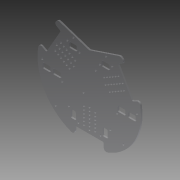
# Autodesk Inventor part: Bottom Plate
Saved by Autodesk Inventor 2015 (Build 190159000, 159)
## iProperties
Created: 2016-02-10
Part Number: Bottom Plate
Material: Polycarbonate, Clear
Document SubType Name: Modeling
Designer: James
Density: 1.2 g/cm^3
Appearance: Polycarbonate - Clear
Mass: 85.2719 g
Surface Area: 524.465 cm^2
Volume: 71.0599 cm^3
Author: James
Autodesk Inventor part; units mm, degrees
ref_plane "YZ Plane" through (0, 0, 0) normal (1, 0, 0) x (0, 1, 0)
ref_plane "XZ Plane" through (0, 0, 0) normal (0, 1, 0) x (-1, 0, 0)
ref_plane "XY Plane" through (0, 0, 0) normal (0, 0, 1) x (1, 0, 0)
sketch "Sketch1" plane through (0, 0, 0) normal (0, 1, 0) x (-1, 0, 0)
  line L0 (69.282, 40) -> (56.282, 62.5167)
  line L1 (69.282, 40) -> (82.282, 17.4833)
  circle A0 centre (63.7395, 36.8) radius 1.65
  circle A1 centre (58.2402, 33.625) radius 1.65
  circle A2 centre (52.7409, 30.45) radius 1.65
  circle A3 centre (47.2417, 27.275) radius 1.65
  circle A4 centre (41.7424, 24.1) radius 1.65
  circle A5 centre (36.2432, 20.925) radius 1.65
  circle A6 centre (30.7439, 17.75) radius 1.65
  circle A7 centre (55.6298, 44.6464) radius 1.65
  circle A8 centre (50.1305, 41.4714) radius 1.65
  circle A9 centre (44.6313, 38.2964) radius 1.65
  circle A10 centre (39.132, 35.1214) radius 1.65
  circle A11 centre (33.6327, 31.9464) radius 1.65
  circle A12 centre (28.1335, 28.7714) radius 1.65
  circle A13 centre (66.4798, 25.8536) radius 1.65
  circle A14 centre (60.9805, 22.6786) radius 1.65
  circle A15 centre (55.4813, 19.5036) radius 1.65
  circle A16 centre (49.982, 16.3286) radius 1.65
  circle A17 centre (44.4827, 13.1536) radius 1.65
  circle A18 centre (38.9835, 9.9786) radius 1.65
  line L2 (57.0141, 65.2487) -> (63.1492, 68.7908)
  line L3 (85.0141, 16.7513) -> (91.1492, 20.2934)
  line L4 (57.4738, 79.1579) -> (1.5811, 60.527)
  line L5 (-1.5811, 60.527) -> (-57.4738, 79.1579)
  line L6 (-69.282, 40) -> (-56.282, 62.5167)
  line L7 (-69.282, 40) -> (-82.282, 17.4833)
  circle A19 centre (-63.7395, 36.8) radius 1.65
  circle A20 centre (-58.2402, 33.625) radius 1.65
  circle A21 centre (-52.7409, 30.45) radius 1.65
  circle A22 centre (-47.2417, 27.275) radius 1.65
  circle A23 centre (-41.7424, 24.1) radius 1.65
  circle A24 centre (-36.2432, 20.925) radius 1.65
  circle A25 centre (-30.7439, 17.75) radius 1.65
  circle A26 centre (-55.6298, 44.6464) radius 1.65
  circle A27 centre (-50.1305, 41.4714) radius 1.65
  circle A28 centre (-44.6313, 38.2964) radius 1.65
  circle A29 centre (-39.132, 35.1214) radius 1.65
  circle A30 centre (-33.6327, 31.9464) radius 1.65
  circle A31 centre (-28.1335, 28.7714) radius 1.65
  circle A32 centre (-66.4798, 25.8536) radius 1.65
  circle A33 centre (-60.9805, 22.6786) radius 1.65
  circle A34 centre (-55.4813, 19.5036) radius 1.65
  circle A35 centre (-49.982, 16.3286) radius 1.65
  circle A36 centre (-44.4827, 13.1536) radius 1.65
  circle A37 centre (-38.9835, 9.9786) radius 1.65
  line L8 (-57.0141, 65.2487) -> (-63.1492, 68.7908)
  line L9 (-85.0141, 16.7513) -> (-91.1492, 20.2934)
  line L10 (0, -80) -> (26, -80)
  line L11 (0, -80) -> (-26, -80)
  circle A38 centre (0, -73.6) radius 1.65
  circle A39 centre (0, -67.25) radius 1.65
  circle A40 centre (0, -60.9) radius 1.65
  circle A41 centre (0, -54.55) radius 1.65
  circle A42 centre (0, -48.2) radius 1.65
  circle A43 centre (0, -41.85) radius 1.65
  circle A44 centre (0, -35.5) radius 1.65
  circle A45 centre (10.85, -70.5) radius 1.65
  circle A46 centre (10.85, -64.15) radius 1.65
  circle A47 centre (10.85, -57.8) radius 1.65
  circle A48 centre (10.85, -51.45) radius 1.65
  circle A49 centre (10.85, -45.1) radius 1.65
  circle A50 centre (10.85, -38.75) radius 1.65
  circle A51 centre (-10.85, -70.5) radius 1.65
  circle A52 centre (-10.85, -64.15) radius 1.65
  circle A53 centre (-10.85, -57.8) radius 1.65
  circle A54 centre (-10.85, -51.45) radius 1.65
  circle A55 centre (-10.85, -45.1) radius 1.65
  circle A56 centre (-10.85, -38.75) radius 1.65
  line L12 (28, -82) -> (28, -89.0842)
  line L13 (-28, -82) -> (-28, -89.0842)
  arc A57 (-62.1631, 78.3311) -> (-63.8413, 76.9694) centre (0, 0) ccw
  arc A58 (-98.5781, 16.8034) -> (-34.7368, -93.7729) centre (0, 0) ccw
  arc A59 (34.7368, -93.7729) -> (98.5781, 16.8034) centre (0, 0) ccw
  arc A60 (63.8413, 76.9694) -> (62.1631, 78.3311) centre (0, 0) ccw
  circle A61 centre (-31.5451, 65.2447) radius 1.6
  circle A62 centre (31.5451, 65.2447) radius 1.6
  circle A63 centre (65.4074, -65.4074) radius 1.6
  circle A64 centre (-65.4074, -65.4074) radius 1.6
  arc A65 (-63.8413, 76.9694) -> (-63.1492, 68.7908) centre (-60.6492, 73.121) ccw
  arc A66 (-57.4738, 79.1579) -> (-62.1631, 78.3311) centre (-59.0549, 74.4145) ccw
  arc A67 (63.1492, 68.7908) -> (63.8413, 76.9694) centre (60.6492, 73.121) ccw
  arc A68 (-91.1492, 20.2934) -> (-98.5781, 16.8034) centre (-93.6492, 15.9633) ccw
  arc A69 (-34.7368, -93.7729) -> (-28, -89.0842) centre (-33, -89.0842) ccw
  arc A70 (28, -89.0842) -> (34.7368, -93.7729) centre (33, -89.0842) ccw
  arc A71 (98.5781, 16.8034) -> (91.1492, 20.2934) centre (93.6492, 15.9633) ccw
  arc A72 (62.1631, 78.3311) -> (57.4738, 79.1579) centre (59.0549, 74.4145) ccw
  arc A73 (-1.5811, 60.527) -> (1.5811, 60.527) centre (0, 65.2705) ccw
  arc A74 (-56.282, 62.5167) -> (-57.0141, 65.2487) centre (-58.0141, 63.5167) ccw
  arc A75 (-85.0141, 16.7513) -> (-82.282, 17.4833) centre (-84.0141, 18.4833) ccw
  arc A76 (-26, -80) -> (-28, -82) centre (-26, -82) ccw
  arc A77 (28, -82) -> (26, -80) centre (26, -82) ccw
  arc A78 (82.282, 17.4833) -> (85.0141, 16.7513) centre (84.0141, 18.4833) ccw
  arc A79 (57.0141, 65.2487) -> (56.282, 62.5167) centre (58.0141, 63.5167) ccw
  line L14 (-25.85, -68.5) -> (-25.85, -57.5)
  line L15 (-27.85, -55.5) -> (-33.85, -55.5)
  line L16 (-35.85, -57.5) -> (-35.85, -68.5)
  line L17 (-33.85, -70.5) -> (-27.85, -70.5)
  arc A80 (-33.85, -55.5) -> (-35.85, -57.5) centre (-33.85, -57.5) ccw
  arc A81 (-25.85, -57.5) -> (-27.85, -55.5) centre (-27.85, -57.5) ccw
  arc A82 (-27.85, -70.5) -> (-25.85, -68.5) centre (-27.85, -68.5) ccw
  arc A83 (-35.85, -68.5) -> (-33.85, -70.5) centre (-33.85, -68.5) ccw
  line L18 (25.85, -68.5) -> (25.85, -57.5)
  arc A84 (25.85, -68.5) -> (27.85, -70.5) centre (27.85, -68.5) ccw
  line L19 (27.85, -55.5) -> (33.85, -55.5)
  arc A85 (27.85, -55.5) -> (25.85, -57.5) centre (27.85, -57.5) ccw
  arc A86 (35.85, -57.5) -> (33.85, -55.5) centre (33.85, -57.5) ccw
  line L20 (35.85, -57.5) -> (35.85, -68.5)
  arc A87 (33.85, -70.5) -> (35.85, -68.5) centre (33.85, -68.5) ccw
  line L21 (33.85, -70.5) -> (27.85, -70.5)
  line L22 (-77, -5) -> (-88, -5)
  arc A88 (-75, -7) -> (-77, -5) centre (-77, -7) ccw
  line L23 (-90, -7) -> (-90, -13)
  arc A89 (-88, -5) -> (-90, -7) centre (-88, -7) ccw
  arc A90 (-90, -13) -> (-88, -15) centre (-88, -13) ccw
  line L24 (-88, -15) -> (-77, -15)
  arc A91 (-77, -15) -> (-75, -13) centre (-77, -13) ccw
  line L25 (-75, -13) -> (-75, -7)
  line L26 (-57, -5) -> (-68, -5)
  arc A92 (-55, -7) -> (-57, -5) centre (-57, -7) ccw
  line L27 (-70, -7) -> (-70, -13)
  arc A93 (-68, -5) -> (-70, -7) centre (-68, -7) ccw
  arc A94 (-70, -13) -> (-68, -15) centre (-68, -13) ccw
  line L28 (-68, -15) -> (-57, -15)
  arc A95 (-57, -15) -> (-55, -13) centre (-57, -13) ccw
  line L29 (-55, -13) -> (-55, -7)
  line L30 (77, -5) -> (88, -5)
  arc A96 (77, -5) -> (75, -7) centre (77, -7) ccw
  line L31 (90, -7) -> (90, -13)
  arc A97 (90, -7) -> (88, -5) centre (88, -7) ccw
  arc A98 (88, -15) -> (90, -13) centre (88, -13) ccw
  line L32 (88, -15) -> (77, -15)
  arc A99 (75, -13) -> (77, -15) centre (77, -13) ccw
  line L33 (75, -13) -> (75, -7)
  line L34 (57, -5) -> (68, -5)
  arc A100 (57, -5) -> (55, -7) centre (57, -7) ccw
  line L35 (70, -7) -> (70, -13)
  arc A101 (70, -7) -> (68, -5) centre (68, -7) ccw
  arc A102 (68, -15) -> (70, -13) centre (68, -13) ccw
  line L36 (68, -15) -> (57, -15)
  arc A103 (55, -13) -> (57, -15) centre (57, -13) ccw
  line L37 (55, -13) -> (55, -7)
  line L38 (-26.0451, 55.2447) -> (-37.0451, 55.2447)
  arc A104 (-24.0451, 53.2447) -> (-26.0451, 55.2447) centre (-26.0451, 53.2447) ccw
  line L39 (-39.0451, 53.2447) -> (-39.0451, 47.2447)
  arc A105 (-37.0451, 55.2447) -> (-39.0451, 53.2447) centre (-37.0451, 53.2447) ccw
  arc A106 (-39.0451, 47.2447) -> (-37.0451, 45.2447) centre (-37.0451, 47.2447) ccw
  line L40 (-37.0451, 45.2447) -> (-26.0451, 45.2447)
  arc A107 (-26.0451, 45.2447) -> (-24.0451, 47.2447) centre (-26.0451, 47.2447) ccw
  line L41 (-24.0451, 47.2447) -> (-24.0451, 53.2447)
  line L42 (37.0451, 55.2447) -> (26.0451, 55.2447)
  arc A108 (39.0451, 53.2447) -> (37.0451, 55.2447) centre (37.0451, 53.2447) ccw
  line L43 (24.0451, 53.2447) -> (24.0451, 47.2447)
  arc A109 (26.0451, 55.2447) -> (24.0451, 53.2447) centre (26.0451, 53.2447) ccw
  arc A110 (24.0451, 47.2447) -> (26.0451, 45.2447) centre (26.0451, 47.2447) ccw
  line L44 (26.0451, 45.2447) -> (37.0451, 45.2447)
  arc A111 (37.0451, 45.2447) -> (39.0451, 47.2447) centre (37.0451, 47.2447) ccw
  line L45 (39.0451, 47.2447) -> (39.0451, 53.2447)
  circle A112 centre (-53.2, -19.3) radius 1.6
  circle A113 centre (-91.8, -0.7) radius 1.6
  circle A114 centre (53.2, -19.3) radius 1.6
  circle A115 centre (91.8, -0.7) radius 1.6
  circle A116 centre (-40.15, -53.7) radius 1.6
  circle A117 centre (-21.55, -72.3) radius 1.6
  circle A118 centre (40.15, -53.7) radius 1.6
  circle A119 centre (21.55, -72.3) radius 1.6
  circle A120 centre (-43.3451, 54.5447) radius 1.6
  circle A121 centre (-19.7451, 45.9447) radius 1.6
  circle A122 centre (43.3451, 54.5447) radius 1.6
  circle A123 centre (19.7451, 45.9447) radius 1.6
  circle A124 centre (11.8, -16.8) radius 1.6
  circle A125 centre (-11.8, 31.8) radius 1.6
  constraints: 126 centre point, 102 point on circle, 92 end point
extrude "Extrusion1" add sketch "Sketch1" along normal blind 3
body "Solid1"
